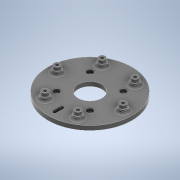
# Autodesk Inventor part: Motorsupport
Saved by Autodesk Inventor 2022 (Build 260153000, 153)
## iProperties
Created: 2022-02-18
Part Number: Motorsupport
Material: Genérico
Document SubType Name: Modeling
Designer: JK
Density: 1 g/cm^3
Appearance: Suave - Negro
Author: JK
Autodesk Inventor part; units mm, degrees
ref_plane "YZ Plane" through (0, 0, 0) normal (1, 0, 0) x (0, 1, 0)
ref_plane "XZ Plane" through (0, 0, 0) normal (0, 1, 0) x (-1, 0, 0)
ref_plane "XY Plane" through (0, 0, 0) normal (0, 0, 1) x (1, 0, 0)
sketch "Boceto1" plane through (0, 0, 0) normal (0, 1, 0) x (-1, 0, 0)
  circle A0 centre (0, 0) radius 11.15
  line L0 (-40, 40) -> (40, 40)
  line L1 (40, 40) -> (40, -40)
  line L2 (40, -40) -> (-40, -40)
  line L3 (-40, -40) -> (-40, 40)
  line L4 (-40, 40) -> (40, -40) construction
  line L5 (40, 40) -> (-40, -40) construction
  dimension "d0" = 22.3
  dimension "d1" = 80
  dimension "d2" = 80
  constraints: 12 end point, 2 midpoint, 2 parallel, 1 centre point, 1 coincident, 1 horizontal, 1 perpendicular
  measures "d0" diameter of A0
  measures "d1" distance of L0.end L1.end
  measures "d2" distance of L1.end L2.end
extrude "Extrusión1" add sketch "Boceto1" along normal blind 4
sketch "Boceto2" plane through (0, 4, 0) normal (0, 1, 0) x (1, 0, 0)
  circle A0 centre (-15.5, -15.5) radius 1.65
  point P0 (0, 0)
  dimension "d5" = 15.5
  dimension "d6" = 15.5
  dimension "d7" = 3.3
  constraints: 1 centre point
  measures "d5" horizontal distance of A0.centre point (0, 0)
  measures "d6" horizontal distance of A0.centre point (0, 0)
  measures "d7" diameter of A0
extrude "Extrusión2" cut sketch "Boceto2" against normal through all
pattern_circular "Patrón circular1" count 4 over 360 about axis through (0, 0, 0) along (0, 1, 0) of "Extrusión2"
chamfer "Chaflán1" distance 1.5 angle 45 4 edges at (-17.15, 4, 15.5) (-15.5, 4, -17.15) (17.15, 4, -15.5) (15.5, 4, 17.15)
sketch "Boceto3" plane through (0, 4, 0) normal (0, 1, 0) x (1, 0, 0)
  circle A0 centre (-30.6, 0) radius 2.925
  point P0 (0, 0)
  dimension "d16" = 5.85
  dimension "d17" = 30.6
  constraints: 1 centre point
  measures "d16" diameter of A0
  measures "d17" distance of point (0, 0) A0.centre
extrude "Extrusión3" add sketch "Boceto3" along normal blind 6
sketch "Boceto4" plane through (0, 4, 0) normal (0, 1, 0) x (1, 0, 0)
  circle A0 centre (-30.6, 0) radius 2.925 projected
  circle A1 centre (-30.6, 0) radius 3.75
  point P0 (0, 0)
  point P1 (-30, -3.9)
  point P2 (-30, 3.9)
  dimension "d20" = 7.5
  constraints: 1 centre point, 1 coincident, 1 other
  measures "d20" diameter of A1
extrude "Extrusión4" add sketch "Boceto4" along normal blind 3 contours A0 | A1
fillet "Empalme1" radius 2 1 edges at (-34.35, 4, 0)
pattern_circular "Patrón circular2" count 6 over 360 about axis through (0, 0, 0) along (0, 1, 0) of "Extrusión3", "Empalme1", "Extrusión4"
sketch "Boceto5" plane through (0, 4, 0) normal (0, 1, 0) x (1, 0, 0)
  circle A0 centre (0, 0) radius 36.5
  circle A1 centre (15.3, 26.5004) radius 5.75 projected
  circle A2 centre (15.3, -26.5004) radius 5.75 projected
  circle A3 centre (-30.6, 0) radius 5.75 projected
  circle A4 centre (15.5, 15.5) radius 3.15 projected
  circle A5 centre (-15.5, -15.5) radius 3.15 projected
  line L0 (40, 40) -> (-40, 40) projected
  line L1 (-40, 40) -> (-40, -40) projected
  line L2 (-40, -40) -> (40, -40) projected
  line L3 (40, -40) -> (40, 40) projected
  circle A6 centre (0, 0) radius 11.15 projected
  circle A7 centre (-15.5, 15.5) radius 3.15 projected
  circle A8 centre (15.5, -15.5) radius 3.15 projected
  circle A9 centre (-15.3, -26.5004) radius 5.75 projected
  circle A10 centre (30.6, 0) radius 5.75 projected
  dimension "d27" = 73
  constraints: 1 centre point, 1 coincident
  measures "d27" diameter of A0
extrude "Extrusión5" cut sketch "Boceto5" against normal through all contours L3 L2 L1 L0
sketch "Boceto6" plane through (0, 4, 0) normal (0, 1, 0) x (1, 0, 0)
  circle A0 centre (0, -33) radius 1.65
  line L0 (-1.65, -33) -> (1.65, -33)
  line L1 (1.65, -33) -> (1.65, -26)
  line L2 (1.65, -26) -> (-1.65, -26)
  line L3 (-1.65, -26) -> (-1.65, -33)
  circle A1 centre (0, -26) radius 1.65
  point P0 (0, 0)
  point P1 (-1.65, -26)
  dimension "d30" = 3.3
  dimension "d31" = 7
  dimension "d32" = 26
  constraints: 8 end point, 2 parallel, 2 vertical, 1 horizontal, 1 midpoint, 1 perpendicular, 1 vertical alignment, 6 other
  measures "d31" distance of L0.end L1.end
  measures "d32" distance of point (0, 0) point (0, -26)
extrude "Extrusión6" cut sketch "Boceto6" against normal through all
sketch "Boceto7" plane through (-30.6, 10, 0) normal (0, 1, 0) x (1, 0, 0)
  circle A0 centre (0, 0) radius 1.6
  point P0 (30.6, 0)
  dimension "d35" = 3.2
  constraints: 1 centre point
  measures "d35" diameter of A0
extrude "Extrusión7" cut sketch "Boceto7" against normal through all
pattern_circular "Patrón circular3" count 6 over 360 about axis through (0, 0, 0) along (0, 1, 0) of "Extrusión7"
sketch "Boceto8" plane through (0, 0, 0) normal (0, -1, 0) x (1, 0, 0)
  circle A0 centre (-15.3, 26.5004) radius 1.6 projected
  circle A1 centre (-15.3, 26.5004) radius 2.85
  line L0 (-12.45, 28.1458) -> (-12.45, 24.8549)
  line L1 (-12.45, 24.8549) -> (-15.3, 23.2095)
  line L2 (-15.3, 23.2095) -> (-18.15, 24.8549)
  line L3 (-18.15, 24.8549) -> (-18.15, 28.1458)
  line L4 (-18.15, 28.1458) -> (-15.3, 29.7913)
  line L5 (-15.3, 29.7913) -> (-12.45, 28.1458)
  line L6 (-24.8914, 27.7755) -> (-11.6086, 35.4444)
  circle A2 centre (0, 0) radius 36.5 projected
  line L7 (-15.3, 26.5004) -> (-18.25, 31.6099)
  dimension "d41" = 5.7
  constraints: 16 end point, 2 coincident, 1 centre point, 1 midpoint, 1 parallel, 1 perpendicular, 1 tangent, 16 other
  measures "d41" diameter of A1
extrude "Extrusión8" [suppressed]
pattern_circular "Patrón circular4" [suppressed]
sketch "Boceto9" plane through (0, 4, 0) normal (0, 1, 0) x (1, 0, 0)
  circle A0 centre (-15.5, -15.5) radius 3.15 projected
  circle A1 centre (-15.5, -15.5) radius 1.65
  point P0 (0, 0)
  dimension "d47" = 3.3
  constraints: 1 centre point, 1 coincident
  measures "d47" diameter of A1
extrude "Extrusión9" add sketch "Boceto9" against normal up to surface (4 mm away)
pattern_circular "Patrón circular5" count 4 over 360 about axis through (0, 0, 0) along (0, 1, 0) of "Extrusión9"
sketch "Boceto10" plane through (0, 4, 0) normal (0, 1, 0) x (1, 0, 0)
  circle A0 centre (-26, 15.0111) radius 2.15
  line L0 (0, 0) -> (-35.1199, 0)
  line L1 (0, 0) -> (-26, 15.0111)
  circle A1 centre (-26, -15.011) radius 2.15
  circle A2 centre (26, 15.0111) radius 2.15
  circle A3 centre (26, -15.011) radius 2.15
  dimension "d53" = 30
  dimension "d54" = 4.3
  dimension "d55" = 26
  dimension "d56" = 26
  dimension "d57" = 15.011
  constraints: 4 centre point, 4 end point, 3 equal radius, 2 horizontal alignment, 2 vertical alignment, 1 horizontal
  measures "d53" angle of L1 L0
  measures "d54" diameter of A0
  measures "d55" horizontal distance of L0.start L1.end
  measures "d56" horizontal distance of L0.start A2.centre
  measures "d57" vertical distance of L0.start A1.centre
extrude "Extrusión10" [suppressed]
sketch "Boceto12" plane through (0, 0, 0) normal (0, -1, 0) x (1, 0, 0)
  circle A0 centre (0, 0) radius 36.5 projected
  circle A1 centre (0, 0) radius 39
  dimension "d61" = 78
  constraints: 1 centre point, 1 coincident
  measures "d61" diameter of A1
extrude "Extrusión11" add sketch "Boceto12" against normal up to surface (4 mm away)
sketch "Boceto13" plane through (0, 4, 0) normal (0, 1, 0) x (1, 0, 0)
  circle A0 centre (-15.5, -15.5) radius 1.65 projected
  circle A1 centre (-15.5, -15.5) radius 2.9
  point P0 (0, 0)
  dimension "d64" = 5.8
  constraints: 1 centre point, 1 coincident
  measures "d64" diameter of A1
extrude "Extrusión12" cut sketch "Boceto13" against normal blind 3 contours A0 | A1
pattern_circular "Patrón circular6" count 4 over 360 about axis through (0, 0, 0) along (0, 1, 0) of "Extrusión12"
